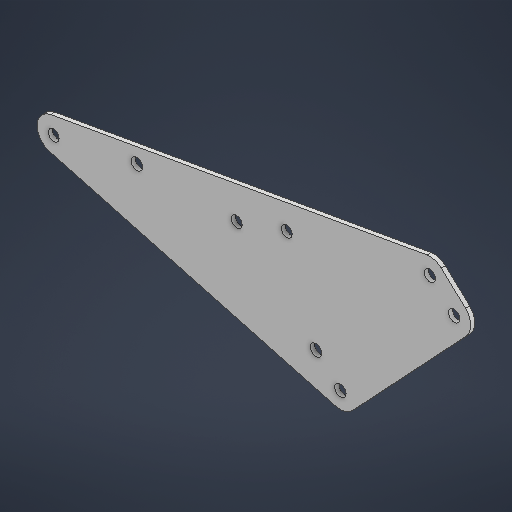
# Autodesk Inventor part: 1-Gearbox
Saved by Autodesk Inventor 2026.1 (Build 301233000, 233)
## iProperties
Created: 2025-08-06
Part Number: 1-Gearbox
Material: Generic
Document SubType Name: Modeling
Designer: roejo
Density: 1 g/cm^3
Appearance: Default
Author: roejo
Autodesk Inventor part; units mm, degrees
ref_plane "YZ Plane" through (0, 0, 0) normal (1, 0, 0) x (0, 1, 0)
ref_plane "XZ Plane" through (0, 0, 0) normal (0, 1, 0) x (-1, 0, 0)
ref_plane "XY Plane" through (0, 0, 0) normal (0, 0, 1) x (1, 0, 0)
sketch "Sketch2" plane through (0, 0, 0) normal (0, 0, 1) x (1, 0, 0)
  circle A0 centre (-58.827, 33.0516) radius 2.1971
  circle A1 centre (-20.727, 33.0516) radius 2.0955
  circle A2 centre (62.1938, 43.4026) radius 2.1844
  circle A3 centre (52.9267, 52.0864) radius 2.1844
  circle A4 centre (18.7744, -2.9332) radius 2.1844
  circle A5 centre (9.5073, 5.7507) radius 2.1844
  circle A6 centre (-90.577, 26.7016) radius 2.0955
  circle A7 centre (-1.677, 39.4016) radius 2.0955
  arc A8 (-91.6831, 32.9546) -> (-92.238, 20.5727) centre (-90.577, 26.7016) ccw
  arc A9 (57.2686, 56.72) -> (51.8206, 58.3394) centre (52.9267, 52.0864) ccw
  arc A10 (66.8274, 39.0606) -> (66.5358, 48.0361) centre (62.1938, 43.4026) ccw
  arc A11 (17.1134, -9.0622) -> (23.408, -7.2752) centre (18.7744, -2.9332) ccw
  line L0 (-92.238, 20.5727) -> (17.1134, -9.0622)
  line L1 (66.8274, 39.0606) -> (23.408, -7.2752)
  line L2 (66.5358, 48.0361) -> (57.2686, 56.72)
  line L3 (51.8206, 58.3394) -> (-91.6831, 32.9546)
  dimension "d17" = 4.191
  dimension "d18" = 4.191
  dimension "d19" = 12.7
  dimension "d20" = 12.7
  dimension "d21" = 12.7
  dimension "d22" = 12.7
  constraints: 12 centre point, 8 end point, 8 point on circle, 7 tangent, 4 coincident, 1 perpendicular, 4 other
  measures "d17" diameter of A6
  measures "d18" diameter of A7
  measures "d19" diameter of A8
  measures "d20" diameter of A9
  measures "d21" diameter of A10
  measures "d22" diameter of A11
extrude "Extrusion2" add sketch "Sketch2" along normal blind 1.5875
body "Solid2"
